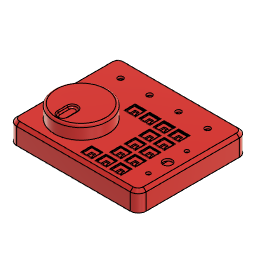
Macropad (Autodesk Fusion 360 design; units mm, degrees)
Autodesk Fusion 360 part; units mm, degrees
(part 1 of 2)
sketch "Sketch1" plane through (0, 0, 0) normal (0, 0, 1) x (1, 0, 0) in component "Top"
  circle A0 centre (0, 0) radius 3.675
  line L0 (80, -25.6) -> (95, -25.6)
  line L1 (95, -25.6) -> (95, -40)
  line L2 (95, -40) -> (80, -40)
  line L3 (80, -40) -> (80, -25.6)
  circle A1 centre (0, 0) radius 37.5
  line L4 (60, -40) -> (60, -25.6)
  line L5 (75, -40) -> (60, -40)
  line L6 (60, -25.6) -> (75, -25.6)
  line L7 (75, -25.6) -> (75, -40)
  line L8 (40, -40) -> (40, -25.6)
  line L9 (55, -40) -> (40, -40)
  line L10 (40, -25.6) -> (55, -25.6)
  line L11 (55, -25.6) -> (55, -40)
  line L12 (80, -20) -> (80, -5.6)
  line L13 (95, -20) -> (80, -20)
  line L14 (80, -5.6) -> (95, -5.6)
  line L15 (95, -5.6) -> (95, -20)
  line L16 (60, -20) -> (60, -5.6)
  line L17 (75, -20) -> (60, -20)
  line L18 (60, -5.6) -> (75, -5.6)
  line L19 (75, -5.6) -> (75, -20)
  line L20 (80, 0) -> (80, 14.4)
  line L21 (95, 0) -> (80, 0)
  line L22 (80, 14.4) -> (95, 14.4)
  line L23 (95, 14.4) -> (95, 0)
  line L24 (60, 0) -> (60, 14.4)
  line L25 (75, 0) -> (60, 0)
  line L26 (60, 14.4) -> (75, 14.4)
  line L27 (75, 14.4) -> (75, 0)
  line L28 (80, 20) -> (80, 34.4)
  line L29 (95, 20) -> (80, 20)
  line L30 (80, 34.4) -> (95, 34.4)
  line L31 (95, 34.4) -> (95, 20)
  line L32 (60, 20) -> (60, 34.4)
  line L33 (75, 20) -> (60, 20)
  line L34 (60, 34.4) -> (75, 34.4)
  line L35 (75, 34.4) -> (75, 20)
  line L36 (80, 40) -> (80, 54.4)
  line L37 (95, 40) -> (80, 40)
  line L38 (80, 54.4) -> (95, 54.4)
  line L39 (95, 54.4) -> (95, 40)
  line L40 (60, 40) -> (60, 54.4)
  line L41 (75, 40) -> (60, 40)
  line L42 (60, 54.4) -> (75, 54.4)
  line L43 (75, 54.4) -> (75, 40)
  line L44 (40, 40) -> (40, 54.4)
  line L45 (55, 40) -> (40, 40)
  line L46 (40, 54.4) -> (55, 54.4)
  line L47 (55, 54.4) -> (55, 40)
  line L48 (20, 40) -> (20, 54.4)
  line L49 (35, 40) -> (20, 40)
  line L50 (20, 54.4) -> (35, 54.4)
  line L51 (35, 54.4) -> (35, 40)
  line L52 (95, 7.2) -> (112, 7.2) construction
  circle A2 centre (112, 7.2) radius 6.25
  line L53 (105.4, 21.75) -> (118.6, 21.75)
  line L54 (118.6, 21.75) -> (118.6, -7.35)
  line L55 (118.6, -7.35) -> (105.4, -7.35)
  line L56 (105.4, -7.35) -> (105.4, 21.75)
  line L57 (112, 21.75) -> (112, -7.35) construction
  line L58 (118.6, 7.2) -> (105.4, 7.2) construction
  circle A3 centre (112, 33.75) radius 2.75
  circle A4 centre (112, -19.35) radius 2.75
  line L59 (112, 21.75) -> (112, 45.3126) construction
  line L60 (0, 0) -> (-50, 0) construction
  circle A5 centre (-20.7, 75) radius 3.675
  circle A6 centre (19.3, 75) radius 3.675
  circle A7 centre (59.3, 75) radius 3.675
  circle A8 centre (99.3, 75) radius 3.675
  line L61 (-50, 92.5) -> (-50, -50)
  line L62 (47.5, -40) -> (47.5, -50) construction
  line L63 (-50, -50) -> (128.6, -50)
  line L64 (118.6, 10.2026) -> (128.6, 10.2026) construction
  line L65 (128.6, -50) -> (128.6, 92.5)
  line L66 (-50, 92.5) -> (128.6, 92.5)
  line L67 (19.3, 75) -> (59.3, 75) construction
  line L68 (39.3, 92.5) -> (39.3, 57.5) construction
  line L69 (-50, 92.5) -> (-50, 100.5)
  line L70 (-50, 100.5) -> (128.6, 100.5)
  line L71 (128.6, 100.5) -> (128.6, 92.5)
  point P0 (112, 7.2)
  dimension "d6" = 7.35
  dimension "d7" = 15
  dimension "d8" = 14.4
  dimension "d9" = 75
  dimension "d10" = 80
  dimension "d13" = -60
  dimension "d14" = 80
  dimension "d17" = 17
  dimension "d18" = 12.5
  dimension "d19" = 29.1
  dimension "d20" = 13.2
  dimension "d21" = 5.5
  dimension "d22" = 12
  dimension "d23" = 40
  dimension "d24" = 7.35
  dimension "d27" = 120
  dimension "d28" = 0
  dimension "d29" = 75
  dimension "d30" = 50
  dimension "d31" = 10
  dimension "d32" = 10
  dimension "d33" = 17.5
  dimension "d88" = 8
  constraint coincident A0.centre A1.centre
  constraint horizontal L0
  constraint vertical L1
  constraint horizontal L2
  constraint vertical L3
  constraint midpoint L23 L52.start
  constraint perpendicular L23 L52
  constraint coincident P0 L52.end
  constraint horizontal L53
  constraint vertical L54
  constraint horizontal L55
  constraint vertical L56
  constraint midpoint L53 L57.start
  constraint midpoint L55 L57.end
  constraint midpoint L54 L58.start
  constraint midpoint L56 L58.end
  constraint midpoint L58 P0
  constraint symmetric L52 A3 A4
  constraint perpendicular L53 L59
  constraint coincident A3.centre L59
  constraint horizontal L60
  constraint vertical L61
  constraint midpoint L9 L62.start
  constraint perpendicular L9 L62
  constraint perpendicular L61 L63
  constraint coincident L54 L64.start
  constraint perpendicular L54 L64
  constraint coincident L63 L65.start
  constraint perpendicular L63 L65
  constraint perpendicular L61 L66
  constraint coincident L65 L66.end
  constraint coincident L62.end L63
  constraint coincident L64.end L65
  constraint coincident A6.centre L67.start
  constraint coincident A7.centre L67.end
  constraint midpoint L66 L68.start
  constraint perpendicular L67 L68
  constraint midpoint L67 L68
  constraint perpendicular L66 L69
  constraint perpendicular L65 L70
  measures "d6" diameter of A0
  measures "d7" distance of L0.start L0.end
  measures "d8" distance of L0.end L1.end
  measures "d9" diameter of A1
  measures "d10" distance of A0.centre L3
  measures "d17" distance of L52.start P0
  measures "d18" diameter of A2
  measures "d19" distance of L53.end L54.end
  measures "d20" distance of L53.start L53.end
  measures "d21" diameter of A3
  measures "d22" distance of L57.start A3.centre
  measures "d23" distance of L2 A0.centre
  measures "d24" diameter of A5
  measures "d29" vertical distance of A0.centre A5.centre
  measures "d30" distance of A0.centre L61
  measures "d31" distance of L62.start L62.end
  measures "d32" distance of L64.start L64.end
  measures "d33" distance of A5.centre L66
  measures "d88" distance of L61.start L69.end
extrude "Extrude1" add sketch "Sketch1" along normal blind 3 contours A1 | L53 L54 L55 L56 | L61 L63 L65 L66 | L66 L69 L70 L71 makes body 1 in component "Top"
sketch "Sketch2" plane through (0, 0, 0) normal (0, 0, -1) x (1, 0, 0) in component "Top"
  line L0 (35, -54.4) -> (20, -54.4)
  line L1 (20, -54.4) -> (20, -40)
  line L2 (20, -40) -> (35, -40)
  line L3 (35, -40) -> (35, -54.4)
  circle A0 centre (112, -33.75) radius 2.75
  circle A1 centre (112, 19.35) radius 2.75
  circle A2 centre (-20.7, -75) radius 3.675
  circle A3 centre (19.3, -75) radius 3.675
  circle A4 centre (59.3, -75) radius 3.675
  circle A5 centre (99.3, -75) radius 3.675
  line L4 (95, -54.4) -> (80, -54.4)
  line L5 (80, -54.4) -> (80, -40)
  line L6 (80, -40) -> (95, -40)
  line L7 (95, -40) -> (95, -54.4)
  line L8 (75, -54.4) -> (60, -54.4)
  line L9 (60, -54.4) -> (60, -40)
  line L10 (60, -40) -> (75, -40)
  line L11 (75, -40) -> (75, -54.4)
  line L12 (55, -54.4) -> (40, -54.4)
  line L13 (40, -54.4) -> (40, -40)
  line L14 (40, -40) -> (55, -40)
  line L15 (55, -40) -> (55, -54.4)
  line L16 (75, -34.4) -> (60, -34.4)
  line L17 (60, -34.4) -> (60, -20)
  line L18 (60, -20) -> (75, -20)
  line L19 (75, -20) -> (75, -34.4)
  line L20 (95, -34.4) -> (80, -34.4)
  line L21 (80, -34.4) -> (80, -20)
  line L22 (80, -20) -> (95, -20)
  line L23 (95, -20) -> (95, -34.4)
  line L24 (75, -14.4) -> (60, -14.4)
  line L25 (60, -14.4) -> (60, 0)
  line L26 (60, 0) -> (75, 0)
  line L27 (75, 0) -> (75, -14.4)
  line L28 (95, -14.4) -> (80, -14.4)
  line L29 (80, -14.4) -> (80, 0)
  line L30 (80, 0) -> (95, 0)
  line L31 (95, 0) -> (95, -14.4)
  line L32 (75, 5.6) -> (60, 5.6)
  line L33 (60, 5.6) -> (60, 20)
  line L34 (60, 20) -> (75, 20)
  line L35 (75, 20) -> (75, 5.6)
  line L36 (95, 5.6) -> (80, 5.6)
  line L37 (80, 5.6) -> (80, 20)
  line L38 (80, 20) -> (95, 20)
  line L39 (95, 20) -> (95, 5.6)
  circle A6 centre (0, 0) radius 3.675
  line L40 (80, 40) -> (95, 40)
  line L41 (95, 40) -> (95, 25.6)
  line L42 (95, 25.6) -> (80, 25.6)
  line L43 (80, 25.6) -> (80, 40)
  line L44 (75, 25.6) -> (60, 25.6)
  line L45 (60, 25.6) -> (60, 40)
  line L46 (60, 40) -> (75, 40)
  line L47 (75, 40) -> (75, 25.6)
  line L48 (55, 25.6) -> (40, 25.6)
  line L49 (40, 25.6) -> (40, 40)
  line L50 (40, 40) -> (55, 40)
  line L51 (55, 40) -> (55, 25.6)
  line L52 (128.6, 50) -> (-50, 50)
  line L53 (-50, 50) -> (-50, -100.5)
  line L54 (128.6, -100.5) -> (128.6, 50)
  line L55 (95.6, 24.75) -> (79.4, 24.75)
  line L56 (79.4, 24.75) -> (79.4, 40.85)
  line L57 (79.4, 40.85) -> (95.6, 40.85)
  line L58 (95.6, 40.85) -> (95.6, 24.75)
  line L59 (95.6, 32.8) -> (79.4, 32.8) construction
  line L60 (87.5, 25.6) -> (87.5, 40) construction
  line L61 (75.6, 24.75) -> (59.4, 24.75)
  line L62 (59.4, 24.75) -> (59.4, 40.85)
  line L63 (59.4, 40.85) -> (75.6, 40.85)
  line L64 (75.6, 40.85) -> (75.6, 24.75)
  line L65 (55.6, 24.75) -> (39.4, 24.75)
  line L66 (39.4, 24.75) -> (39.4, 40.85)
  line L67 (39.4, 40.85) -> (55.6, 40.85)
  line L68 (55.6, 40.85) -> (55.6, 24.75)
  line L69 (95.6, 4.75) -> (79.4, 4.75)
  line L70 (79.4, 4.75) -> (79.4, 20.85)
  line L71 (79.4, 20.85) -> (95.6, 20.85)
  line L72 (95.6, 20.85) -> (95.6, 4.75)
  line L73 (75.6, 4.75) -> (59.4, 4.75)
  line L74 (59.4, 4.75) -> (59.4, 20.85)
  line L75 (59.4, 20.85) -> (75.6, 20.85)
  line L76 (75.6, 20.85) -> (75.6, 4.75)
  line L77 (95.6, -15.25) -> (79.4, -15.25)
  line L78 (79.4, -15.25) -> (79.4, 0.85)
  line L79 (79.4, 0.85) -> (95.6, 0.85)
  line L80 (95.6, 0.85) -> (95.6, -15.25)
  line L81 (75.6, -15.25) -> (59.4, -15.25)
  line L82 (59.4, -15.25) -> (59.4, 0.85)
  line L83 (59.4, 0.85) -> (75.6, 0.85)
  line L84 (75.6, 0.85) -> (75.6, -15.25)
  line L85 (95.6, -35.25) -> (79.4, -35.25)
  line L86 (79.4, -35.25) -> (79.4, -19.15)
  line L87 (79.4, -19.15) -> (95.6, -19.15)
  line L88 (95.6, -19.15) -> (95.6, -35.25)
  line L89 (75.6, -35.25) -> (59.4, -35.25)
  line L90 (59.4, -35.25) -> (59.4, -19.15)
  line L91 (59.4, -19.15) -> (75.6, -19.15)
  line L92 (75.6, -19.15) -> (75.6, -35.25)
  line L93 (95.6, -55.25) -> (79.4, -55.25)
  line L94 (79.4, -55.25) -> (79.4, -39.15)
  line L95 (79.4, -39.15) -> (95.6, -39.15)
  line L96 (95.6, -39.15) -> (95.6, -55.25)
  line L97 (75.6, -55.25) -> (59.4, -55.25)
  line L98 (59.4, -55.25) -> (59.4, -39.15)
  line L99 (59.4, -39.15) -> (75.6, -39.15)
  line L100 (75.6, -39.15) -> (75.6, -55.25)
  line L101 (55.6, -55.25) -> (39.4, -55.25)
  line L102 (39.4, -55.25) -> (39.4, -39.15)
  line L103 (39.4, -39.15) -> (55.6, -39.15)
  line L104 (55.6, -39.15) -> (55.6, -55.25)
  line L105 (35.6, -55.25) -> (19.4, -55.25)
  line L106 (19.4, -55.25) -> (19.4, -39.15)
  line L107 (19.4, -39.15) -> (35.6, -39.15)
  line L108 (35.6, -39.15) -> (35.6, -55.25)
  circle A7 centre (112, -7.2) radius 6.25
  line L109 (-50, -100.5) -> (128.6, -100.5)
  dimension "d36" = 16.1
  dimension "d37" = 16.2
  dimension "d40" = -60
  dimension "d41" = -80
  constraint horizontal L55
  constraint vertical L56
  constraint horizontal L57
  constraint vertical L58
  constraint midpoint L58 L59.start
  constraint midpoint L56 L59.end
  constraint midpoint L42 L60.start
  constraint midpoint L40 L60.end
  constraint midpoint L59 L60
  measures "d36" distance of L55.start L57.end
  measures "d37" distance of L55.start L55.end
extrude "Extrude2" cut sketch "Sketch2" against normal blind 2.1 contours L55 L56 L57 L58 | L61 L62 L63 L64 | L65 L66 L67 L68 | L69 L70 L71 L72 | L73 L74 L75 L76 | L77 L78 L79 L80 | L81 L82 L83 L84 | L85 L86 L87 L88 | L89 L90 L91 L92 | L93 L94 L95 L96 | L97 L98 L99 L100 | L101 L102 L103 L104 | L105 L106 L107 L108 bodies 1 in component "Top"
ref_plane "WorkPlane1" through (39.3, 25.25, -4.4) normal (0, 0, -1) x (-1, 0, 0) in component "Top"
sketch "Sketch3" plane through (39.025, 21.25, -4.4) normal (0, 0, -1) x (1, 0, 0) in component "Top"
  line L0 (55.975, -18.75) -> (40.975, -18.75)
  line L1 (55.975, -33.15) -> (55.975, -18.75)
  line L2 (40.975, -33.15) -> (55.975, -33.15)
  line L3 (40.975, -18.75) -> (40.975, -33.15)
  line L4 (48.475, -18.75) -> (48.475, -21.75)
  line L5 (48.475, -21.75) -> (51.475, -21.75)
  line L6 (51.475, -21.75) -> (51.475, -27.95)
  line L7 (51.475, -27.95) -> (46.375, -27.95)
  line L8 (46.375, -27.95) -> (46.375, -33.15)
  line L9 (54.375, -18.75) -> (54.375, -20.35)
  line L10 (54.375, -20.35) -> (55.975, -20.35)
  line L11 (54.375, -18.75) -> (48.475, -18.75)
  line L12 (54.375, -33.15) -> (54.375, -31.55)
  line L13 (54.375, -31.55) -> (55.975, -31.55)
  line L14 (54.375, -18.75) -> (55.975, -18.75)
  line L15 (55.975, -20.35) -> (55.975, -18.75)
  line L16 (54.375, -33.15) -> (55.975, -33.15)
  line L17 (55.975, -31.55) -> (55.975, -33.15)
  line L18 (-24.1636, -37.438) -> (59.2594, -37.438)
  line L19 (62.4135, -20.9371) -> (62.4135, 48.3711)
  line L20 (62.4135, 66.891) -> (-24.1636, 66.891)
  line L21 (-24.1636, 66.891) -> (-24.1636, -37.438)
  line L22 (62.4135, -20.9371) -> (82.1047, -20.9371)
  line L23 (82.1047, -20.9371) -> (82.1047, -44.9617)
  line L24 (82.1047, -44.9617) -> (59.2594, -44.9617)
  line L25 (59.2594, -44.9617) -> (59.2594, -37.438)
  line L26 (62.4135, 66.891) -> (82.6632, 66.891)
  line L27 (82.6632, 66.891) -> (82.6632, 48.3711)
  line L28 (82.6632, 48.3711) -> (62.4135, 48.3711)
  line L29 (34.375, -20.35) -> (35.975, -20.35)
  line L30 (35.975, -18.75) -> (20.975, -18.75)
  line L31 (28.475, -21.75) -> (31.475, -21.75)
  line L32 (31.475, -27.95) -> (26.375, -27.95)
  line L33 (26.375, -27.95) -> (26.375, -33.15)
  line L34 (28.475, -18.75) -> (28.475, -21.75)
  line L35 (34.375, -18.75) -> (35.975, -18.75)
  line L36 (35.975, -31.55) -> (35.975, -33.15)
  line L37 (34.375, -18.75) -> (28.475, -18.75)
  line L38 (31.475, -21.75) -> (31.475, -27.95)
  line L39 (35.975, -20.35) -> (35.975, -18.75)
  line L40 (34.375, -18.75) -> (34.375, -20.35)
  line L41 (20.975, -33.15) -> (35.975, -33.15)
  line L42 (35.975, -33.15) -> (35.975, -18.75)
  line L43 (34.375, -33.15) -> (35.975, -33.15)
  line L44 (34.375, -31.55) -> (35.975, -31.55)
  line L45 (34.375, -33.15) -> (34.375, -31.55)
  line L46 (20.975, -18.75) -> (20.975, -33.15)
  line L47 (14.375, -20.35) -> (15.975, -20.35)
  line L48 (15.975, -18.75) -> (0.975, -18.75)
  line L49 (8.475, -21.75) -> (11.475, -21.75)
  line L50 (11.475, -27.95) -> (6.375, -27.95)
  line L51 (6.375, -27.95) -> (6.375, -33.15)
  line L52 (8.475, -18.75) -> (8.475, -21.75)
  line L53 (14.375, -18.75) -> (15.975, -18.75)
  line L54 (15.975, -31.55) -> (15.975, -33.15)
  line L55 (14.375, -18.75) -> (8.475, -18.75)
  line L56 (11.475, -21.75) -> (11.475, -27.95)
  line L57 (15.975, -20.35) -> (15.975, -18.75)
  line L58 (14.375, -18.75) -> (14.375, -20.35)
  line L59 (0.975, -33.15) -> (15.975, -33.15)
  line L60 (15.975, -33.15) -> (15.975, -18.75)
  line L61 (14.375, -33.15) -> (15.975, -33.15)
  line L62 (14.375, -31.55) -> (15.975, -31.55)
  line L63 (14.375, -33.15) -> (14.375, -31.55)
  line L64 (0.975, -18.75) -> (0.975, -33.15)
  line L65 (-5.625, -20.35) -> (-4.025, -20.35)
  line L66 (-4.025, -18.75) -> (-19.025, -18.75)
  line L67 (-11.525, -21.75) -> (-8.525, -21.75)
  line L68 (-8.525, -27.95) -> (-13.625, -27.95)
  line L69 (-13.625, -27.95) -> (-13.625, -33.15)
  line L70 (-11.525, -18.75) -> (-11.525, -21.75)
  line L71 (-5.625, -18.75) -> (-4.025, -18.75)
  line L72 (-4.025, -31.55) -> (-4.025, -33.15)
  line L73 (-5.625, -18.75) -> (-11.525, -18.75)
  line L74 (-8.525, -21.75) -> (-8.525, -27.95)
  line L75 (-4.025, -20.35) -> (-4.025, -18.75)
  line L76 (-5.625, -18.75) -> (-5.625, -20.35)
  line L77 (-19.025, -33.15) -> (-4.025, -33.15)
  line L78 (-4.025, -33.15) -> (-4.025, -18.75)
  line L79 (-5.625, -33.15) -> (-4.025, -33.15)
  line L80 (-5.625, -31.55) -> (-4.025, -31.55)
  line L81 (-5.625, -33.15) -> (-5.625, -31.55)
  line L82 (-19.025, -18.75) -> (-19.025, -33.15)
  line L83 (54.375, -0.35) -> (55.975, -0.35)
  line L84 (55.975, 1.25) -> (40.975, 1.25)
  line L85 (48.475, -1.75) -> (51.475, -1.75)
  line L86 (51.475, -7.95) -> (46.375, -7.95)
  line L87 (46.375, -7.95) -> (46.375, -13.15)
  line L88 (48.475, 1.25) -> (48.475, -1.75)
  line L89 (54.375, 1.25) -> (55.975, 1.25)
  line L90 (55.975, -11.55) -> (55.975, -13.15)
  line L91 (54.375, 1.25) -> (48.475, 1.25)
  line L92 (51.475, -1.75) -> (51.475, -7.95)
  line L93 (55.975, -0.35) -> (55.975, 1.25)
  line L94 (54.375, 1.25) -> (54.375, -0.35)
  line L95 (40.975, -13.15) -> (55.975, -13.15)
  line L96 (55.975, -13.15) -> (55.975, 1.25)
  line L97 (54.375, -13.15) -> (55.975, -13.15)
  line L98 (54.375, -11.55) -> (55.975, -11.55)
  line L99 (54.375, -13.15) -> (54.375, -11.55)
  line L100 (40.975, 1.25) -> (40.975, -13.15)
  line L101 (34.375, -0.35) -> (35.975, -0.35)
  line L102 (35.975, 1.25) -> (20.975, 1.25)
  line L103 (28.475, -1.75) -> (31.475, -1.75)
  line L104 (31.475, -7.95) -> (26.375, -7.95)
  line L105 (26.375, -7.95) -> (26.375, -13.15)
  line L106 (28.475, 1.25) -> (28.475, -1.75)
  line L107 (34.375, 1.25) -> (35.975, 1.25)
  line L108 (35.975, -11.55) -> (35.975, -13.15)
  line L109 (34.375, 1.25) -> (28.475, 1.25)
  line L110 (31.475, -1.75) -> (31.475, -7.95)
  line L111 (35.975, -0.35) -> (35.975, 1.25)
  line L112 (34.375, 1.25) -> (34.375, -0.35)
  line L113 (20.975, -13.15) -> (35.975, -13.15)
  line L114 (35.975, -13.15) -> (35.975, 1.25)
  line L115 (34.375, -13.15) -> (35.975, -13.15)
  line L116 (34.375, -11.55) -> (35.975, -11.55)
  line L117 (34.375, -13.15) -> (34.375, -11.55)
  line L118 (20.975, 1.25) -> (20.975, -13.15)
  line L119 (54.375, 19.65) -> (55.975, 19.65)
  line L120 (55.975, 21.25) -> (40.975, 21.25)
  line L121 (48.475, 18.25) -> (51.475, 18.25)
  line L122 (51.475, 12.05) -> (46.375, 12.05)
  line L123 (46.375, 12.05) -> (46.375, 6.85)
  line L124 (48.475, 21.25) -> (48.475, 18.25)
  line L125 (54.375, 21.25) -> (55.975, 21.25)
  line L126 (55.975, 8.45) -> (55.975, 6.85)
  line L127 (54.375, 21.25) -> (48.475, 21.25)
  line L128 (51.475, 18.25) -> (51.475, 12.05)
  line L129 (55.975, 19.65) -> (55.975, 21.25)
  line L130 (54.375, 21.25) -> (54.375, 19.65)
  line L131 (40.975, 6.85) -> (55.975, 6.85)
  line L132 (55.975, 6.85) -> (55.975, 21.25)
  line L133 (54.375, 6.85) -> (55.975, 6.85)
  line L134 (54.375, 8.45) -> (55.975, 8.45)
  line L135 (54.375, 6.85) -> (54.375, 8.45)
  line L136 (40.975, 21.25) -> (40.975, 6.85)
  line L137 (34.375, 19.65) -> (35.975, 19.65)
  line L138 (35.975, 21.25) -> (20.975, 21.25)
  line L139 (28.475, 18.25) -> (31.475, 18.25)
  line L140 (31.475, 12.05) -> (26.375, 12.05)
  line L141 (26.375, 12.05) -> (26.375, 6.85)
  line L142 (28.475, 21.25) -> (28.475, 18.25)
  line L143 (34.375, 21.25) -> (35.975, 21.25)
  line L144 (35.975, 8.45) -> (35.975, 6.85)
  line L145 (34.375, 21.25) -> (28.475, 21.25)
  line L146 (31.475, 18.25) -> (31.475, 12.05)
  line L147 (35.975, 19.65) -> (35.975, 21.25)
  line L148 (34.375, 21.25) -> (34.375, 19.65)
  line L149 (20.975, 6.85) -> (35.975, 6.85)
  line L150 (35.975, 6.85) -> (35.975, 21.25)
  line L151 (34.375, 6.85) -> (35.975, 6.85)
  line L152 (34.375, 8.45) -> (35.975, 8.45)
  line L153 (34.375, 6.85) -> (34.375, 8.45)
  line L154 (20.975, 21.25) -> (20.975, 6.85)
  line L155 (54.375, 39.65) -> (55.975, 39.65)
  line L156 (55.975, 41.25) -> (40.975, 41.25)
  line L157 (48.475, 38.25) -> (51.475, 38.25)
  line L158 (51.475, 32.05) -> (46.375, 32.05)
  line L159 (46.375, 32.05) -> (46.375, 26.85)
  line L160 (48.475, 41.25) -> (48.475, 38.25)
  line L161 (54.375, 41.25) -> (55.975, 41.25)
  line L162 (55.975, 28.45) -> (55.975, 26.85)
  line L163 (54.375, 41.25) -> (48.475, 41.25)
  line L164 (51.475, 38.25) -> (51.475, 32.05)
  line L165 (55.975, 39.65) -> (55.975, 41.25)
  line L166 (54.375, 41.25) -> (54.375, 39.65)
  line L167 (40.975, 26.85) -> (55.975, 26.85)
  line L168 (55.975, 26.85) -> (55.975, 41.25)
  line L169 (54.375, 26.85) -> (55.975, 26.85)
  line L170 (54.375, 28.45) -> (55.975, 28.45)
  line L171 (54.375, 26.85) -> (54.375, 28.45)
  line L172 (40.975, 41.25) -> (40.975, 26.85)
  line L173 (34.375, 39.65) -> (35.975, 39.65)
  line L174 (35.975, 41.25) -> (20.975, 41.25)
  line L175 (28.475, 38.25) -> (31.475, 38.25)
  line L176 (31.475, 32.05) -> (26.375, 32.05)
  line L177 (26.375, 32.05) -> (26.375, 26.85)
  line L178 (28.475, 41.25) -> (28.475, 38.25)
  line L179 (34.375, 41.25) -> (35.975, 41.25)
  line L180 (35.975, 28.45) -> (35.975, 26.85)
  line L181 (34.375, 41.25) -> (28.475, 41.25)
  line L182 (31.475, 38.25) -> (31.475, 32.05)
  line L183 (35.975, 39.65) -> (35.975, 41.25)
  line L184 (34.375, 41.25) -> (34.375, 39.65)
  line L185 (20.975, 26.85) -> (35.975, 26.85)
  line L186 (35.975, 26.85) -> (35.975, 41.25)
  line L187 (34.375, 26.85) -> (35.975, 26.85)
  line L188 (34.375, 28.45) -> (35.975, 28.45)
  line L189 (34.375, 26.85) -> (34.375, 28.45)
  line L190 (20.975, 41.25) -> (20.975, 26.85)
  line L191 (54.375, 59.65) -> (55.975, 59.65)
  line L192 (55.975, 61.25) -> (40.975, 61.25)
  line L193 (48.475, 58.25) -> (51.475, 58.25)
  line L194 (51.475, 52.05) -> (46.375, 52.05)
  line L195 (46.375, 52.05) -> (46.375, 46.85)
  line L196 (48.475, 61.25) -> (48.475, 58.25)
  line L197 (54.375, 61.25) -> (55.975, 61.25)
  line L198 (55.975, 48.45) -> (55.975, 46.85)
  line L199 (54.375, 61.25) -> (48.475, 61.25)
  line L200 (51.475, 58.25) -> (51.475, 52.05)
  line L201 (55.975, 59.65) -> (55.975, 61.25)
  line L202 (54.375, 61.25) -> (54.375, 59.65)
  line L203 (40.975, 46.85) -> (55.975, 46.85)
  line L204 (55.975, 46.85) -> (55.975, 61.25)
  line L205 (54.375, 46.85) -> (55.975, 46.85)
  line L206 (54.375, 48.45) -> (55.975, 48.45)
  line L207 (54.375, 46.85) -> (54.375, 48.45)
  line L208 (40.975, 61.25) -> (40.975, 46.85)
  line L209 (34.375, 59.65) -> (35.975, 59.65)
  line L210 (35.975, 61.25) -> (20.975, 61.25)
  line L211 (28.475, 58.25) -> (31.475, 58.25)
  line L212 (31.475, 52.05) -> (26.375, 52.05)
  line L213 (26.375, 52.05) -> (26.375, 46.85)
  line L214 (28.475, 61.25) -> (28.475, 58.25)
  line L215 (34.375, 61.25) -> (35.975, 61.25)
  line L216 (35.975, 48.45) -> (35.975, 46.85)
  line L217 (34.375, 61.25) -> (28.475, 61.25)
  line L218 (31.475, 58.25) -> (31.475, 52.05)
  line L219 (35.975, 59.65) -> (35.975, 61.25)
  line L220 (34.375, 61.25) -> (34.375, 59.65)
  line L221 (20.975, 46.85) -> (35.975, 46.85)
  line L222 (35.975, 46.85) -> (35.975, 61.25)
  line L223 (34.375, 46.85) -> (35.975, 46.85)
  line L224 (34.375, 48.45) -> (35.975, 48.45)
  line L225 (34.375, 46.85) -> (34.375, 48.45)
  line L226 (20.975, 61.25) -> (20.975, 46.85)
  line L227 (14.375, 59.65) -> (15.975, 59.65)
  line L228 (15.975, 61.25) -> (0.975, 61.25)
  line L229 (8.475, 58.25) -> (11.475, 58.25)
  line L230 (11.475, 52.05) -> (6.375, 52.05)
  line L231 (6.375, 52.05) -> (6.375, 46.85)
  line L232 (8.475, 61.25) -> (8.475, 58.25)
  line L233 (14.375, 61.25) -> (15.975, 61.25)
  line L234 (15.975, 48.45) -> (15.975, 46.85)
  line L235 (14.375, 61.25) -> (8.475, 61.25)
  line L236 (11.475, 58.25) -> (11.475, 52.05)
  line L237 (15.975, 59.65) -> (15.975, 61.25)
  line L238 (14.375, 61.25) -> (14.375, 59.65)
  line L239 (0.975, 46.85) -> (15.975, 46.85)
  line L240 (15.975, 46.85) -> (15.975, 61.25)
  line L241 (14.375, 46.85) -> (15.975, 46.85)
  line L242 (14.375, 48.45) -> (15.975, 48.45)
  line L243 (14.375, 46.85) -> (14.375, 48.45)
  line L244 (0.975, 61.25) -> (0.975, 46.85)
  dimension "d45" = 3
  dimension "d46" = 3
  dimension "d47" = 6.2
  dimension "d48" = 1.6
  dimension "d49" = 1.6
  dimension "d50" = 1.6
  dimension "d51" = 1.6
  dimension "d58" = 8
  dimension "d161" = -60
  dimension "d162" = 80
  constraint midpoint L0 L4.start
  constraint perpendicular L0 L4
  constraint perpendicular L4 L5
  constraint perpendicular L5 L6
  constraint perpendicular L6 L7
  constraint perpendicular L2 L8
  constraint perpendicular L0 L9
  constraint coincident L1 L10.end
  constraint perpendicular L1 L10
  constraint perpendicular L4 L11
  constraint coincident L2 L12.start
  constraint perpendicular L2 L12
  constraint coincident L1 L13.end
  constraint perpendicular L1 L13
  constraint coincident L0.start L1.end
  constraint coincident L1.start L2.end
  constraint horizontal L18
  constraint vertical L19
  constraint horizontal L20
  constraint vertical L21
  constraint perpendicular L19 L22
  constraint perpendicular L22 L23
  constraint perpendicular L19 L24
  constraint perpendicular L18 L25
  constraint perpendicular L19 L26
  constraint perpendicular L26 L27
  constraint perpendicular L19 L28
  constraint coincident L2 L8.end
  measures "d45" distance of L4.start L4.end
  measures "d46" distance of L4.end L5.end
  measures "d47" distance of L5.end L6.end
  measures "d48" distance of L0.start L9.start
  measures "d49" distance of L9.start L9.end
  measures "d50" distance of L12.start L12.end
  measures "d51" distance of L12.end L13.end
  measures "d58" distance of L8.end L12.start
extrude "Extrude5" add sketch "Sketch3" along normal blind 2 separate body contours L0 L1 L2 L4 L5 L6 L7 L8 L9 L10 L11 L12 L13 | L18 L19 L20 L21 L22 L23 L24 L25 L26 L27 L28 | L29 L30 L31 L32 L33 L34 L37 L38 L40 L41 L42 L44 L45 | L47 L48 L49 L50 L51 L52 L55 L56 L58 L59 L60 L62 L63 | L65 L66 L67 L68 L69 L70 L73 L74 L76 L77 L78 L80 L81 | L83 L84 L85 L86 L87 L88 L91 L92 L94 L95 L96 L98 L99 | L101 L102 L103 L104 L105 L106 L109 L110 L112 L113 L114 L116 L117 | L119 L120 L121 L122 L123 L124 L127 L128 L130 L131 L132 L134 L135 | L137 L138 L139 L140 L141 L142 L145 L146 L148 L149 L150 L152 L153 | L155 L156 L157 L158 L159 L160 L163 L164 L166 L167 L168 L170 L171 | L173 L174 L175 L176 L177 L178 L181 L182 L184 L185 L186 L188 L189 | L191 L192 L193 L194 L195 L196 L199 L200 L202 L203 L204 L206 L207 | L209 L210 L211 L212 L213 L214 L217 L218 L220 L221 L222 L224 L225 | L227 L228 L229 L230 L231 L232 L235 L236 L238 L239 L240 L242 L243 makes body 2 in component "Top"
copy_body "Body->Comp1" bodies 2 removing the originals makes body 3 in component "Holding Plate"
sketch "Sketch6" plane through (0, 0, 0) normal (0, 0, -1) x (1, 0, 0) in component "Top"
  line L0 (59.4, -55.25) -> (59.4, -39.15)
  line L1 (59.4, -39.15) -> (75.6, -39.15)
  line L2 (75.6, -39.15) -> (75.6, -55.25)
  line L3 (75.6, -55.25) -> (59.4, -55.25)
  line L4 (59.4, -15.25) -> (59.4, 0.85)
  line L5 (59.4, 0.85) -> (75.6, 0.85)
  line L6 (75.6, 0.85) -> (75.6, -15.25)
  line L7 (75.6, -15.25) -> (59.4, -15.25)
  line L8 (39.4, 24.75) -> (39.4, 40.85)
  line L9 (39.4, 40.85) -> (55.6, 40.85)
  line L10 (55.6, 40.85) -> (55.6, 24.75)
  line L11 (55.6, 24.75) -> (39.4, 24.75)
  line L12 (59.4, 24.75) -> (59.4, 40.85)
  line L13 (59.4, 40.85) -> (75.6, 40.85)
  line L14 (75.6, 40.85) -> (75.6, 24.75)
  line L15 (75.6, 24.75) -> (59.4, 24.75)
  line L16 (79.4, -15.25) -> (79.4, 0.85)
  line L17 (79.4, 0.85) -> (95.6, 0.85)
  line L18 (95.6, 0.85) -> (95.6, -15.25)
  line L19 (95.6, -15.25) -> (79.4, -15.25)
  line L20 (79.4, -55.25) -> (79.4, -39.15)
  line L21 (79.4, -39.15) -> (95.6, -39.15)
  line L22 (95.6, -39.15) -> (95.6, -55.25)
  line L23 (95.6, -55.25) -> (79.4, -55.25)
  line L24 (39.4, -55.25) -> (39.4, -39.15)
  line L25 (39.4, -39.15) -> (55.6, -39.15)
  line L26 (55.6, -39.15) -> (55.6, -55.25)
  line L27 (55.6, -55.25) -> (39.4, -55.25)
  line L28 (79.4, -35.25) -> (79.4, -19.15)
  line L29 (79.4, -19.15) -> (95.6, -19.15)
  line L30 (95.6, -19.15) -> (95.6, -35.25)
  line L31 (95.6, -35.25) -> (79.4, -35.25)
  line L32 (59.4, 4.75) -> (59.4, 20.85)
  line L33 (59.4, 20.85) -> (75.6, 20.85)
  line L34 (75.6, 20.85) -> (75.6, 4.75)
  line L35 (75.6, 4.75) -> (59.4, 4.75)
  line L36 (79.4, 24.75) -> (79.4, 40.85)
  line L37 (79.4, 40.85) -> (95.6, 40.85)
  line L38 (95.6, 40.85) -> (95.6, 24.75)
  line L39 (95.6, 24.75) -> (79.4, 24.75)
  line L40 (79.4, 4.75) -> (79.4, 20.85)
  line L41 (79.4, 20.85) -> (95.6, 20.85)
  line L42 (95.6, 20.85) -> (95.6, 4.75)
  line L43 (95.6, 4.75) -> (79.4, 4.75)
  line L44 (59.4, -35.25) -> (59.4, -19.15)
  line L45 (59.4, -19.15) -> (75.6, -19.15)
  line L46 (75.6, -19.15) -> (75.6, -35.25)
  line L47 (75.6, -35.25) -> (59.4, -35.25)
  line L48 (19.4, -55.25) -> (19.4, -39.15)
  line L49 (19.4, -39.15) -> (35.6, -39.15)
  line L50 (35.6, -39.15) -> (35.6, -55.25)
  line L51 (35.6, -55.25) -> (19.4, -55.25)
  circle A0 centre (0, 0) radius 3.675
  circle A1 centre (59.3, -75) radius 3.675
  circle A2 centre (-20.7, -75) radius 3.675
  circle A3 centre (19.3, -75) radius 3.675
  circle A4 centre (99.3, -75) radius 3.675
  circle A5 centre (112, 19.35) radius 2.75
  circle A6 centre (112, -7.2) radius 6.25
  circle A7 centre (112, -33.75) radius 2.75
  line L52 (128.6, 50) -> (-50, 50)
  line L53 (-50, 50) -> (-50, -100.5)
  line L54 (128.6, -100.5) -> (128.6, 50)
  line L55 (128.6, -56.2797) -> (123.6, -56.2797) construction
  line L56 (78.805, -100.5) -> (78.805, -97.5) construction
  line L57 (-50, -34.1893) -> (-44, -34.1893) construction
  line L58 (40.2828, 50) -> (40.2828, 46.8) construction
  line L59 (-44, 46.8) -> (123.05, 46.8)
  line L60 (123.05, 46.8) -> (123.05, -97.5)
  line L61 (123.05, -97.5) -> (-44, -97.5)
  line L62 (-44, -97.5) -> (-44, 46.8)
  line L63 (-50, -100.5) -> (128.6, -100.5)
  dimension "d81" = 5
  dimension "d82" = 3
  dimension "d83" = 6
  dimension "d84" = 3.2
  constraint coincident L54 L55.start
  constraint perpendicular L54 L55
  constraint coincident L53 L57.start
  constraint perpendicular L53 L57
  constraint coincident L52 L58.start
  constraint perpendicular L52 L58
  constraint perpendicular L54 L59
  constraint perpendicular L55 L60
  constraint perpendicular L53 L61
  constraint perpendicular L59 L62
  constraint coincident L56.start L63
  constraint coincident L56.end L61
  constraint coincident L58.end L59
  measures "d81" distance of L55.start L55.end
  measures "d82" distance of L56.start L56.end
  measures "d83" distance of L57.start L57.end
  measures "d84" distance of L58.start L58.end
extrude "Extrude8" add sketch "Sketch6" along normal blind 24 contours L52 L53 L54 L63 bodies 1 in component "Top"
sketch "Sketch7" plane through (0, 0, 0) normal (0, 0, -1) x (1, 0, 0) in component "Top"
  line L0 (123.05, -97.5) -> (123.05, 46.8)
  line L1 (123.05, 46.8) -> (-44, 46.8)
  line L2 (-44, 46.8) -> (-44, -97.5)
  line L3 (-44, -97.5) -> (123.05, -97.5)
  line L4 (59.4, -55.25) -> (59.4, -39.15)
  line L5 (59.4, -39.15) -> (75.6, -39.15)
  line L6 (75.6, -39.15) -> (75.6, -55.25)
  line L7 (75.6, -55.25) -> (59.4, -55.25)
  line L8 (59.4, -15.25) -> (59.4, 0.85)
  line L9 (59.4, 0.85) -> (75.6, 0.85)
  line L10 (75.6, 0.85) -> (75.6, -15.25)
  line L11 (75.6, -15.25) -> (59.4, -15.25)
  line L12 (39.4, 24.75) -> (39.4, 40.85)
  line L13 (55.6, 40.85) -> (55.6, 24.75)
  line L14 (55.6, 24.75) -> (39.4, 24.75)
  line L15 (59.4, 24.75) -> (59.4, 40.85)
  line L16 (75.6, 40.85) -> (75.6, 24.75)
  line L17 (75.6, 24.75) -> (59.4, 24.75)
  line L18 (79.4, -15.25) -> (79.4, 0.85)
  line L19 (79.4, 0.85) -> (95.6, 0.85)
  line L20 (95.6, 0.85) -> (95.6, -15.25)
  line L21 (95.6, -15.25) -> (79.4, -15.25)
  line L22 (79.4, -55.25) -> (79.4, -39.15)
  line L23 (79.4, -39.15) -> (95.6, -39.15)
  line L24 (95.6, -39.15) -> (95.6, -55.25)
  line L25 (95.6, -55.25) -> (79.4, -55.25)
  line L26 (39.4, -55.25) -> (39.4, -39.15)
  line L27 (39.4, -39.15) -> (55.6, -39.15)
  line L28 (55.6, -39.15) -> (55.6, -55.25)
  line L29 (55.6, -55.25) -> (39.4, -55.25)
  line L30 (79.4, -35.25) -> (79.4, -19.15)
  line L31 (79.4, -19.15) -> (95.6, -19.15)
  line L32 (95.6, -19.15) -> (95.6, -35.25)
  line L33 (95.6, -35.25) -> (79.4, -35.25)
  line L34 (59.4, 4.75) -> (59.4, 20.85)
  line L35 (59.4, 20.85) -> (75.6, 20.85)
  line L36 (75.6, 20.85) -> (75.6, 4.75)
  line L37 (75.6, 4.75) -> (59.4, 4.75)
  line L38 (79.4, 24.75) -> (79.4, 40.85)
  line L39 (95.6, 40.85) -> (95.6, 24.75)
  line L40 (95.6, 24.75) -> (79.4, 24.75)
  line L41 (79.4, 4.75) -> (79.4, 20.85)
  line L42 (79.4, 20.85) -> (95.6, 20.85)
  line L43 (95.6, 20.85) -> (95.6, 4.75)
  line L44 (95.6, 4.75) -> (79.4, 4.75)
  line L45 (59.4, -35.25) -> (59.4, -19.15)
  line L46 (59.4, -19.15) -> (75.6, -19.15)
  line L47 (75.6, -19.15) -> (75.6, -35.25)
  line L48 (75.6, -35.25) -> (59.4, -35.25)
  line L49 (19.4, -55.25) -> (19.4, -39.15)
  line L50 (19.4, -39.15) -> (35.6, -39.15)
  line L51 (35.6, -39.15) -> (35.6, -55.25)
  line L52 (35.6, -55.25) -> (19.4, -55.25)
  circle A0 centre (0, 0) radius 3.675
  circle A1 centre (59.3, -75) radius 3.675
  circle A2 centre (-20.7, -75) radius 3.675
  circle A3 centre (19.3, -75) radius 3.675
  circle A4 centre (99.3, -75) radius 3.675
  circle A5 centre (112, 19.35) radius 2.75
  circle A6 centre (112, -7.2) radius 6.25
  circle A7 centre (112, -33.75) radius 2.75
  line L53 (39.4, 40.85) -> (55.6, 40.85)
  line L54 (59.4, 40.85) -> (75.6, 40.85)
  line L55 (79.4, 40.85) -> (95.6, 40.85)
  line L56 (39.525, -97.5) -> (39.525, -75.5) construction
  line L57 (39.525, -75.5) -> (30.425, -75.5)
  line L58 (30.425, -75.5) -> (30.425, -97.5)
  line L59 (48.625, -75.5) -> (48.625, -97.5)
  line L60 (39.525, -75.5) -> (48.625, -75.5)
  line L61 (48.625, -78.9971) -> (51.625, -78.9971) construction
  line L62 (51.475, -97.5) -> (51.475, -75.5)
  line L63 (51.475, -75.5) -> (48.625, -75.5)
  line L64 (27.575, -97.5) -> (27.575, -75.5)
  line L65 (27.575, -75.5) -> (30.425, -75.5)
  line L66 (27.575, -97.5) -> (30.425, -97.5)
  line L67 (48.625, -97.5) -> (51.475, -97.5)
  dimension "d91" = 22
  dimension "d92" = 9.1
  dimension "d93" = 3
  constraint midpoint L3 L56.start
  constraint perpendicular L3 L56
  constraint perpendicular L56 L57
  constraint coincident L3 L58.end
  constraint perpendicular L3 L58
  constraint symmetric L57.start L56 L60.start
  constraint symmetric L56 L57.end L59.start
  constraint symmetric L56 L58.end L59.end
  constraint coincident L59 L61.start
  constraint perpendicular L59 L61
  constraint coincident L3 L62.start
  constraint perpendicular L60 L62
  constraint perpendicular L59 L63
  constraint symmetric L56 L59.start L57.end
  constraint symmetric L56 L62.start L64.start
  constraint symmetric L56 L62.end L64.end
  constraint perpendicular L58 L66
  measures "d91" distance of L56.start L56.end
  measures "d92" distance of L56.end L57.end
  measures "d93" distance of L61.start L61.end
extrude "Extrude9" add sketch "Sketch7" along normal blind 4 contours L3 L59 L62 L63 L67 | L3 L58 L64 L65 L66 bodies 1 in component "Top"
sketch "Sketch8" plane through (0, 97.5, 0) normal (0, -1, 0) x (1, 0, 0) in component "Top"
  line L0 (51.475, 0) -> (51.475, -4)
  line L1 (51.475, -4) -> (48.625, -4)
  line L2 (48.625, -4) -> (48.625, 0)
  line L3 (48.625, 0) -> (30.425, 0)
  line L4 (30.425, 0) -> (30.425, -4)
  line L5 (30.425, -4) -> (27.575, -4)
  line L6 (27.575, -4) -> (27.575, 0)
  line L7 (27.575, 0) -> (-44, 0)
  line L8 (-44, 0) -> (-44, -24)
  line L9 (-44, -24) -> (123.05, -24)
  line L10 (123.05, -24) -> (123.05, 0)
  line L11 (123.05, 0) -> (51.475, 0)
  line L12 (30.425, -4) -> (31.925, -6.5981)
  line L13 (30.425, -4) -> (33.575, -4) construction
  line L14 (31.925, -6.5981) -> (27.575, -6.5981)
  line L15 (27.575, -6.5981) -> (27.575, -4)
  line L16 (48.625, -4) -> (47.125, -6.5981)
  line L17 (47.125, -6.5981) -> (51.475, -6.5981)
  line L18 (51.475, -6.5981) -> (51.475, -4)
  line L19 (39.525, 0) -> (48.625, 0) construction
  line L20 (39.525, 0) -> (45.025, 0)
  line L21 (39.525, 0) -> (34.025, 0)
  line L22 (34.025, 0) -> (34.025, -7.2)
  line L23 (34.025, -7.2) -> (45.025, -7.2)
  line L24 (45.025, -7.2) -> (45.025, 0)
  line L25 (34.025, -1) -> (45.025, -1)
  dimension "d96" = 3
  dimension "d97" = 60
  dimension "d98" = 3
  dimension "d101" = 120
  dimension "d104" = 5.5
  dimension "d105" = 5.5
  dimension "d106" = 7.2
  dimension "d174" = 1
  constraint horizontal L13
  constraint coincident L4.end L5.start
  constraint perpendicular L6 L14
  constraint coincident L5.end L6.start
  constraint perpendicular L5 L15
  constraint coincident L1.end L2.start
  constraint perpendicular L0 L17
  constraint coincident L0.end L1.start
  constraint perpendicular L1 L18
  constraint midpoint L3 L19.start
  constraint coincident L2.end L3.start
  constraint parallel L3 L20
  constraint parallel L3 L21
  constraint perpendicular L3 L22
  constraint perpendicular L22 L23
  constraint perpendicular L3 L24
  constraint coincident L22 L25.start
  constraint coincident L24 L25.end
  constraint perpendicular L24 L25
  measures "d96" distance of L4.end L12.end
  measures "d97" angle of L12 L13
  measures "d98" distance of L1.end L16.end
  measures "d101" angle of L1 L16
  measures "d104" distance of L19.start L20.end
  measures "d105" distance of L19.start L21.end
  measures "d106" distance of L21.end L22.end
  measures "d174" distance of L20 L25
extrude "Extrude11" cut sketch "Sketch8" against normal blind 3 contours L22 L23 L24 L25 bodies 1 in component "Top"
sketch "Sketch1 (2)" plane through (0, 0, 3) normal (0, 0, 1) x (-1, 0, 0) in component "Big Wheel"
  circle A0 centre (-112, -33.75) radius 2.75
  circle A1 centre (-112, 19.35) radius 2.75
  circle A2 centre (20.7, -75) radius 3.675
  circle A3 centre (-19.3, -75) radius 3.675
  circle A4 centre (-112, -7.2) radius 6.25
  line L0 (-20, -54.4) -> (-35, -54.4)
  line L1 (-35, -54.4) -> (-35, -40)
  line L2 (-35, -40) -> (-20, -40)
  line L3 (-20, -40) -> (-20, -54.4)
  line L4 (-40, -54.4) -> (-55, -54.4)
  line L5 (-55, -54.4) -> (-55, -40)
  line L6 (-55, -40) -> (-40, -40)
  line L7 (-40, -40) -> (-40, -54.4)
  line L8 (-60, -54.4) -> (-75, -54.4)
  line L9 (-75, -54.4) -> (-75, -40)
  line L10 (-75, -40) -> (-60, -40)
  line L11 (-60, -40) -> (-60, -54.4)
  line L12 (-80, -54.4) -> (-95, -54.4)
  line L13 (-95, -54.4) -> (-95, -40)
  line L14 (-95, -40) -> (-80, -40)
  line L15 (-80, -40) -> (-80, -54.4)
  line L16 (-60, -34.4) -> (-75, -34.4)
  line L17 (-75, -34.4) -> (-75, -20)
  line L18 (-75, -20) -> (-60, -20)
  line L19 (-60, -20) -> (-60, -34.4)
  line L20 (-80, -14.4) -> (-95, -14.4)
  line L21 (-95, -14.4) -> (-95, 0)
  line L22 (-95, 0) -> (-80, 0)
  line L23 (-80, 0) -> (-80, -14.4)
  line L24 (-60, -14.4) -> (-75, -14.4)
  line L25 (-75, -14.4) -> (-75, 0)
  line L26 (-75, 0) -> (-60, 0)
  line L27 (-60, 0) -> (-60, -14.4)
  line L28 (-80, -34.4) -> (-95, -34.4)
  line L29 (-95, -34.4) -> (-95, -20)
  line L30 (-95, -20) -> (-80, -20)
  line L31 (-80, -20) -> (-80, -34.4)
  circle A5 centre (0, 0) radius 3.675
  line L32 (-95, 40) -> (-80, 40)
  line L33 (-80, 40) -> (-80, 25.6)
  line L34 (-80, 25.6) -> (-95, 25.6)
  line L35 (-95, 25.6) -> (-95, 40)
  line L36 (-60, 25.6) -> (-75, 25.6)
  line L37 (-75, 25.6) -> (-75, 40)
  line L38 (-75, 40) -> (-60, 40)
  line L39 (-60, 40) -> (-60, 25.6)
  line L40 (-80, 5.6) -> (-95, 5.6)
  line L41 (-95, 5.6) -> (-95, 20)
  line L42 (-95, 20) -> (-80, 20)
  line L43 (-80, 20) -> (-80, 5.6)
  line L44 (-60, 5.6) -> (-75, 5.6)
  line L45 (-75, 5.6) -> (-75, 20)
  line L46 (-75, 20) -> (-60, 20)
  line L47 (-60, 20) -> (-60, 5.6)
  line L48 (-40, 25.6) -> (-55, 25.6)
  line L49 (-55, 25.6) -> (-55, 40)
  line L50 (-55, 40) -> (-40, 40)
  line L51 (-40, 40) -> (-40, 25.6)
  circle A6 centre (-99.3, -75) radius 3.675
  circle A7 centre (-59.3, -75) radius 3.675
  line L52 (50, -100.5) -> (50, 50)
  line L53 (50, 50) -> (-128.6, 50)
  line L54 (-128.6, 50) -> (-128.6, -100.5)
  line L55 (-128.6, -100.5) -> (50, -100.5)
  circle A8 centre (0, 0) radius 37
  dimension "d111" = 74
  constraint coincident A5.centre A8.centre
  measures "d111" diameter of A8
extrude "Extrude1'" add sketch "Sketch1 (2)" along normal blind 13 separate body contours A5 | A8 makes body 4 in component "Big Wheel"
sketch "Sketch2 (2)" plane through (0, 0, 16) normal (0, 0, 1) x (-1, 0, 0) in component "Big Wheel"
  circle A0 centre (0, 0) radius 37
  line L0 (0, 31.4036) -> (0, 6.4036) construction
  line L1 (0, 6.4036) -> (6, 6.4036)
  line L2 (0, 6.4036) -> (-6, 6.4036)
  line L3 (-6, 6.4036) -> (-6, 31.4036)
  line L4 (-6, 31.4036) -> (6, 31.4036)
  line L5 (6, 31.4036) -> (6, 6.4036)
  dimension "d114" = 25
  dimension "d115" = 6
  dimension "d116" = 6
  constraint vertical L0
  constraint perpendicular L0 L1
  constraint perpendicular L0 L2
  constraint perpendicular L2 L3
  constraint perpendicular L3 L4
  constraint perpendicular L1 L5
  measures "d114" distance of L0.start L0.end
  measures "d115" distance of L0.end L1.end
  measures "d116" distance of L0.end L2.end
extrude "Extrude2'" cut sketch "Sketch2 (2)" against normal blind 3 contours L1 L2 L3 L4 L5 bodies 4 in component "Big Wheel"
fillet "Fillet1" radius 6 4 edges at (-6, -6.4036, 14.5) (6, -6.4036, 14.5) (-6, -31.4036, 14.5) (6, -31.4036, 14.5) on bodies 4 in component "Big Wheel"
fillet "Fillet2" radius 1.5 4 edges at (-6, -18.9036, 16) (0, -6.4036, 16) (6, -18.9036, 16) (0, -31.4036, 16) on bodies 4 in component "Big Wheel"
fillet "Fillet3" radius 2 4 edges at (-6, -18.9036, 13) (0, -31.4036, 13) (6, -18.9036, 13) (0, -6.4036, 13) on bodies 4 in component "Big Wheel"
fillet "Fillet4" radius 3 1 edges at (34.4961, 13.3798, 16) on bodies 4 in component "Big Wheel"
sketch "Sketch3 (2)" plane through (0, 0, 3) normal (0, 0, -1) x (1, 0, 0) in component "Big Wheel"
  circle A0 centre (0, 0) radius 37
  line L0 (-2.2373, 1.9987) -> (2.2626, 1.9699)
  arc A1 (-2.2373, 1.9987) -> (2.2626, 1.9699) centre (0, 0) ccw
  arc A2 (-2.3331, 2.2193) -> (2.3613, 2.1893) centre (0, 0) ccw
  line L1 (-2.3331, 2.2193) -> (2.3613, 2.1893)
  dimension "d127" = 6
  dimension "d128" = 4.5
  dimension "d175" = 0.22
  constraint coincident A0.centre A1.centre
  measures "d127" diameter of A1
  measures "d128" distance of L0.start L0.end
extrude "Extrude3" cut sketch "Sketch3 (2)" against normal blind 10.2 contours L0 A1 | A2 L1 bodies 4 in component "Big Wheel"
fillet "Fillet1'" radius 11 4 edges at (-50, -50, -10.5) (128.6, -50, -10.5) (128.6, 100.5, -10.5) (-50, 100.5, -10.5) on bodies 1 in component "Top"
chamfer "Chamfer2" distance 4 angle 45 8 edges at (39.3, 100.5, 3) (-46.7782, 97.2782, 3) (-50, 25.25, 3) (-46.7782, -46.7782, 3) (39.3, -50, 3) (125.3782, -46.7782, 3) (128.6, 25.25, 3) (125.3782, 97.2782, 3) on bodies 1 in component "Top"
fillet "Fillet4'" radius 10 4 edges at (-44, -46.8, -12) (-44, 97.5, -12) (123.05, 97.5, -12) (123.05, -46.8, -12) on bodies 1 in component "Top"
fillet "Fillet1''" radius 9.5 1 edges at (121.6882, -45.641, -5.4) on bodies 3 in component "Holding Plate"
fillet "Fillet5" radius 0.5 4 edges at (34.025, 99, -7.2) (45.025, 99, -7.2) (34.025, 99, -1) (45.025, 99, -1) on bodies 1 in component "Top"
ref_plane "WorkPlane1" through (39.3, 25.25, -21) normal (0, 0, -1) x (-1, 0, 0) in component "Base"
sketch "Sketch1 (3)" plane through (39.025, 25.25, -21) normal (0, 0, -1) x (1, 0, 0) in component "Base"
  line L0 (-83.025, -62.25) -> (-83.025, 62.05)
  arc A0 (-73.025, 72.05) -> (-83.025, 62.05) centre (-73.025, 62.05) ccw
  line L1 (-73.025, 72.05) -> (74.025, 72.05)
  arc A1 (84.025, 62.05) -> (74.025, 72.05) centre (74.025, 62.05) ccw
  line L2 (84.025, 62.05) -> (84.025, -62.25)
  arc A2 (74.025, -72.25) -> (84.025, -62.25) centre (74.025, -62.25) ccw
  line L3 (74.025, -72.25) -> (-73.025, -72.25)
  arc A3 (-83.025, -62.25) -> (-73.025, -72.25) centre (-73.025, -62.25) ccw
  line L4 (-73.025, 71.85) -> (74.025, 71.85)
  arc A4 (83.825, 62.05) -> (74.025, 71.85) centre (74.025, 62.05) ccw
  line L5 (83.825, 62.05) -> (83.825, -62.25)
  arc A5 (74.025, -72.05) -> (83.825, -62.25) centre (74.025, -62.25) ccw
  line L6 (74.025, -72.05) -> (-73.025, -72.05)
  arc A6 (-82.825, -62.25) -> (-73.025, -72.05) centre (-73.025, -62.25) ccw
  line L7 (-82.825, -62.25) -> (-82.825, 62.05)
  arc A7 (-73.025, 71.85) -> (-82.825, 62.05) centre (-73.025, 62.05) ccw
  dimension "d151" = -0.2
extrude "Extrude1''" add sketch "Sketch1 (3)" along normal blind 3 separate body contours L4 A4 L5 A5 L6 A6 L7 A7 makes body 5 in component "Base"
ref_plane "WorkPlane2" through (39.3, 25.25, -21) normal (0, 0, -1) x (-1, 0, 0) in component "Top"
sketch "Sketch10" plane through (39.025, 25.25, -21) normal (0, 0, -1) x (1, 0, 0) in component "Top"
  line L0 (-83.025, -62.25) -> (-83.025, 62.05)
  arc A0 (-83.025, -62.25) -> (-73.025, -72.25) centre (-73.025, -62.25) ccw
  line L1 (74.025, -72.25) -> (-73.025, -72.25)
  arc A1 (74.025, -72.25) -> (84.025, -62.25) centre (74.025, -62.25) ccw
  line L2 (84.025, 62.05) -> (84.025, -62.25)
  arc A2 (84.025, 62.05) -> (74.025, 72.05) centre (74.025, 62.05) ccw
  line L3 (-73.025, 72.05) -> (74.025, 72.05)
  arc A3 (-73.025, 72.05) -> (-83.025, 62.05) centre (-73.025, 62.05) ccw
  arc A4 (-81.025, -62.25) -> (-73.025, -70.25) centre (-73.025, -62.25) ccw
  line L4 (74.025, -70.25) -> (-73.025, -70.25)
  arc A5 (74.025, -70.25) -> (82.025, -62.25) centre (74.025, -62.25) ccw
  line L5 (82.025, 62.05) -> (82.025, -62.25)
  arc A6 (82.025, 62.05) -> (74.025, 70.05) centre (74.025, 62.05) ccw
  line L6 (-73.025, 70.05) -> (74.025, 70.05)
  arc A7 (-73.025, 70.05) -> (-81.025, 62.05) centre (-73.025, 62.05) ccw
  line L7 (-81.025, -62.25) -> (-81.025, 62.05)
  dimension "d155" = 2
extrude "Extrude13" add sketch "Sketch10" against normal blind 1 bodies 1 in component "Top"
chamfer "Chamfer1" distance 2 angle 45 8 edges at (-44, 25.35, -20) (-41.0711, 94.5711, -20) (39.525, 97.5, -20) (120.1211, 94.5711, -20) (123.05, 25.35, -20) (120.1211, -43.8711, -20) (39.525, -46.8, -20) (-41.0711, -43.8711, -20) on bodies 1 in component "Top"